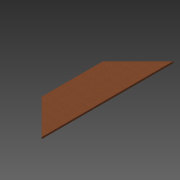
# Autodesk Inventor part: top long
Saved by Autodesk Inventor 2015 (Build 190159000, 159)
## iProperties
Created: 2019-04-10
Part Number: top long
Material: Generic
Document SubType Name: Modeling
Designer: Raptor
Density: 1 g/cm^3
Appearance: English Oak
Author: Raptor
Autodesk Inventor part; units mm, degrees
ref_plane "YZ Plane" through (0, 0, 0) normal (1, 0, 0) x (0, 1, 0)
ref_plane "XZ Plane" through (0, 0, 0) normal (0, 1, 0) x (-1, 0, 0)
ref_plane "XY Plane" through (0, 0, 0) normal (0, 0, 1) x (1, 0, 0)
sketch "Sketch4" plane through (0, 0, 0) normal (0, 1, 0) x (-1, 0, 0)
  line L0 (0, 0) -> (0, -1500)
  line L1 (0, -1500) -> (400, -1100)
  line L2 (400, -1100) -> (400, -400)
  line L3 (400, -400) -> (0, 0)
  dimension "d5" = 45
  dimension "d6" = 45
  dimension "d7" = 700
  dimension "d8" = 1500
  constraints: 8 end point, 1 parallel, 1 vertical
  measures "d5" angle of L3 L0
  measures "d6" angle of L1 L0
  measures "d7" distance of L1.end L2.end
  measures "d8" distance of L0.start L0.end
extrude "Extrusion1" add sketch "Sketch4" along normal blind 20
body "Solid1"
